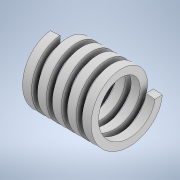
# Autodesk Inventor part: Spirala
Saved by Autodesk Inventor 2021 (Build 250183000, 183)
## iProperties
Created: 2020-04-11
Part Number: Spirala
Material: Ogólny
Document SubType Name: Modeling
Designer: dyrag
Density: 1 g/cm^3
Appearance: Domyślna
Author: dyrag
Autodesk Inventor part; units mm, degrees
ref_plane "YZ Plane" through (0, 0, 0) normal (1, 0, 0) x (0, 1, 0)
ref_plane "XZ Plane" through (0, 0, 0) normal (0, 1, 0) x (-1, 0, 0)
ref_plane "XY Plane" through (0, 0, 0) normal (0, 0, 1) x (1, 0, 0)
ref_plane "Płaszczyzna konstrukcyjna1" through (57.707219, -33.461709, -20.176016) normal (0.081831, 0.9965675, 0.0125239) x (-0.9966457, 0.0818374, 0)
sketch "Szkic2" plane through (57.707219, -33.461709, -20.176016) normal (0.081831, 0.9965675, 0.0125239) x (-0.9966457, 0.0818374, 0)
  line L0 (3, -2) -> (-3, -2)
  line L1 (-3, -2) -> (-3, 3)
  line L2 (-3, 3) -> (3, 3)
  line L3 (3, 3) -> (3, -2)
  point P0 (60.252071, 19.815913)
  constraints: 8 end point, 2 parallel, 1 horizontal, 1 perpendicular
sketch3d "Szkic 3D1"
  helix H0 starts at (10.187219, -14.32129, -0.793546) axis through (10.187219, -33.70529, -0.793546) along (1, 0, 0) pitch 10 turns 4.752 hand right
sweep "Przeciągnięcie1" add profiles "Szkic2" path "Szkic 3D1"
